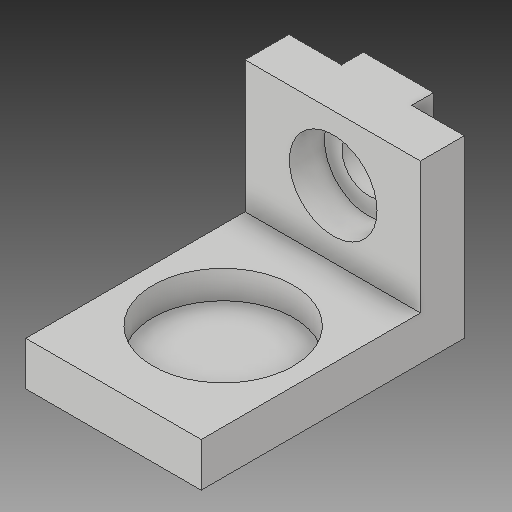
# Autodesk Inventor part: spring tab for on arm
Saved by Autodesk Inventor 2019 (Build 230136000, 136)
## iProperties
Created: 2019-10-26
Part Number: spring tab for on arm
Material: Generic
Document SubType Name: Modeling
Designer: User
Density: 1 g/cm^3
Appearance: Default
Author: User
Autodesk Inventor part; units mm, degrees
ref_plane "YZ Plane" through (0, 0, 0) normal (1, 0, 0) x (0, 1, 0)
ref_plane "XZ Plane" through (0, 0, 0) normal (0, 1, 0) x (-1, 0, 0)
ref_plane "XY Plane" through (0, 0, 0) normal (0, 0, 1) x (1, 0, 0)
sketch "Sketch1" plane through (0, 0, 0) normal (1, 0, 0) x (0, 1, 0)
  line L0 (0, 0) -> (0, -19.05)
  line L1 (0, -19.05) -> (12.7, -19.05)
  line L2 (12.7, -19.05) -> (12.7, -15.875)
  line L3 (12.7, -15.875) -> (3.175, -15.875)
  line L4 (3.175, -15.875) -> (3.175, 0)
  line L5 (3.175, 0) -> (0, 0)
  dimension "d0" = 3.175
  dimension "d1" = 12.7
  dimension "d4" = 3.175
  dimension "d5" = 19.05
  constraints: 12 end point, 4 perpendicular, 2 vertical
  measures "d0" distance of L1.end L2.end
  measures "d1" distance of L0.end L1.end
  measures "d4" distance of L4.end L0.start
  measures "d5" distance of L0.start L0.end
extrude "Extrusion1" add sketch "Sketch1" along normal blind 12.7
sketch "Sketch3" plane through (0, 3.175, 0) normal (0, 1, 0) x (1, 0, 0)
  line L0 (0, 15.875) -> (0, 0) projected
  line L1 (0, 0) -> (12.7, 0) projected
  line L2 (12.7, 15.875) -> (12.7, 0) projected
  line L3 (0, 15.875) -> (12.7, 15.875) projected
  point P0 (0, 0)
  point P1 (6.35, 7.9375)
hole "Hole2" at (6.35, 3.175, -7.9375) direction (0, -1, 0) diameter 10.16 depth 2.032
sketch "Sketch4" plane through (0, 0, -19.05) normal (0, 0, -1) x (-1, 0, 0)
  line L0 (0, 12.7) -> (-12.7, 12.7) projected
  line L1 (0, 0) -> (-12.7, 0) projected
  line L2 (-8.89, 12.7) -> (-3.81, 12.7)
  line L3 (-3.81, 12.7) -> (-3.81, 0)
  line L4 (-3.81, 0) -> (-8.89, 0)
  line L5 (-8.89, 0) -> (-8.89, 12.7)
  line L6 (0, 0) -> (0, 12.7) projected
  line L7 (0, 12.7) -> (-12.7, 12.7) projected
  line L8 (-12.7, 0) -> (-12.7, 12.7) projected
  line L9 (0, 0) -> (-12.7, 0) projected
  dimension "d22" = 5.08
  dimension "d23" = 12.7
  dimension "d24" = 3.81
  constraints: 8 end point, 2 parallel, 2 point on line, 1 horizontal, 1 perpendicular
  measures "d22" distance between parallel lines of L3 L5
  measures "d23" distance between parallel lines of L6 L8
  measures "d24" distance between parallel lines of L6 L3
extrude "Extrusion2" add sketch "Sketch4" along normal blind 1.5875 contours L3 L1 L5 L0
sketch "Sketch5" plane through (0, 3.175, -15.875) normal (0, 0, 1) x (1, 0, 0)
  line L0 (0, 9.525) -> (0, 0) projected
  line L1 (0, 0) -> (12.7, 0) projected
  line L2 (12.7, 9.525) -> (12.7, 0) projected
  line L3 (0, 9.525) -> (12.7, 9.525) projected
  point P0 (0, -3.175)
  point P1 (6.3842, 4.8389)
hole "Hole3" at (6.3842, 8.0139, -15.875) direction (0, 0, -1) diameter 3.81 end through all counterbore diameter 6.35 counterbore depth 2.54
equation "\"d4\" = d0"
equation "\"d24\" = -0.5 * d22 + 0.5 * d23"
body "Solid1"
